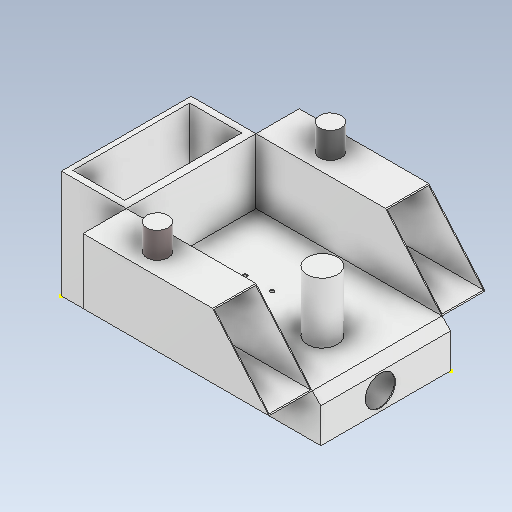
# Autodesk Inventor part: Body
Saved by Autodesk Inventor 2021 (Build 250183000, 183)
## iProperties
Created: 2021-07-15
Part Number: Body
Material: Acetal Resin, White
Document SubType Name: Modeling
Designer: HP
Density: 1.425 g/cm^3
Appearance: Smooth - White
Author: HP
Autodesk Inventor part; units mm, degrees
ref_plane "YZ Plane" through (0, 0, 0) normal (1, 0, 0) x (0, 1, 0)
ref_plane "XZ Plane" through (0, 0, 0) normal (0, 1, 0) x (-1, 0, 0)
sketch "Sketch1" plane through (0, 0, 0) normal (0, 0, 1) x (1, 0, 0)
  line L0 (0, 0) -> (300, 0)
  line L1 (300, 0) -> (300, 50)
  line L2 (300, 50) -> (0, 50)
  line L3 (0, 50) -> (0, 0)
  dimension "d0" = 300
  dimension "d1" = 50
  constraints: 8 end point, 2 parallel, 1 horizontal, 1 perpendicular
  measures "d0" distance of L2.end L1.end
  measures "d1" distance of L0.end L1.end
extrude "Extrusion1" add sketch "Sketch1" along normal blind 150
sketch "Sketch2" plane through (0, 50, 0) normal (0, 1, 0) x (1, 0, 0)
  line L0 (0, 0) -> (0, -150) projected
  line L1 (300, -150) -> (0, -150) projected
  line L2 (0, 0) -> (75, 0)
  line L3 (75, 0) -> (75, -150)
  line L4 (75, -150) -> (0, -150)
  line L5 (0, -150) -> (0, 0)
  line L6 (5.9297, -7.65) -> (65.9297, -7.65)
  line L7 (65.9297, -7.65) -> (65.9297, -142.65)
  line L8 (65.9297, -142.65) -> (5.9297, -142.65)
  line L9 (5.9297, -142.65) -> (5.9297, -7.65)
  dimension "d4" = 75
  dimension "d5" = 60
  dimension "d6" = 135
  dimension "d7" = 7.35
  constraints: 16 end point, 4 parallel, 2 horizontal, 2 perpendicular, 1 point on line
  measures "d4" distance of L3.end L4.end
  measures "d5" distance of L7.end L8.end
  measures "d6" distance of L6.end L7.end
  measures "d7" distance between parallel lines of L8 L1
extrude "Extrusion2" add sketch "Sketch2" along normal blind 75
sketch "Sketch3" plane through (300, 50, 150) normal (0, 1, 0) x (1, 0, 0)
  point P0 (-300, 150)
chamfer "Chamfer1" distance 10 angle 45 1 edges at (300, 50, 75)
sketch "Sketch5" plane through (75, 50, 150) normal (1, 0, 0) x (0, 0, -1)
  point P0 (150, -50)
sketch "Sketch6" plane through (0, 0, 150) normal (0, 0, 1) x (1, 0, 0)
  line L0 (75, 125) -> (224.8279, 125)
  line L1 (290, 50) -> (75, 50) projected
  line L2 (224.8279, 125) -> (290, 50)
  line L3 (75, 125) -> (75, 50)
  line L4 (290, 50) -> (75, 50) projected
  line L5 (75, 50) -> (290, 50)
  point P0 (0, 0)
  constraints: 8 end point, 1 collinear, 1 horizontal
extrude "Extrusion4" add sketch "Sketch6" along normal blind 50
sketch "Sketch7" plane through (0, 0, 150) normal (0, 0, -1) x (-1, 0, 0)
  point P0 (0, 0)
sketch "Sketch8" plane through (0, 0, 0) normal (0, 0, -1) x (-1, 0, 0)
  line L0 (-224.8279, 125) -> (-75, 125) projected
  line L1 (-75, 125) -> (-224.8279, 125)
  line L2 (-290, 50) -> (-300, 40) projected
  line L3 (-224.8279, 125) -> (-290, 50)
  line L4 (-290, 50) -> (-75, 50)
  line L5 (0, 125) -> (-75, 125) projected
  line L6 (-75, 50) -> (-75, 125)
  point P0 (0, 0)
  constraints: 8 end point, 1 collinear, 1 parallel, 1 perpendicular
extrude "Extrusion5" add sketch "Sketch8" along normal blind 50
shell "Shell1" thickness 1 removed faces 2 at (268.276, 75, 183.3333) at (246.5519, 100, -33.3333)
sketch "Sketch9" plane through (75, 125, 150) normal (0, 1, 0) x (1, 0, 0)
  circle A0 centre (61.0187, -25) radius 12.5
  circle A1 centre (61.0187, 175) radius 12.5
  circle A2 centre (61.0187, -29.8112) radius 0.5
  circle A3 centre (61.0187, -24.9762) radius 0.5
  point P0 (-75, 150)
  dimension "d22" = 25
  dimension "d23" = 25
  dimension "d32" = 1
  dimension "d33" = 1
  dimension "d34" = 4.835
  constraints: 4 centre point
  measures "d22" diameter of A0
  measures "d23" diameter of A1
  measures "d32" diameter of A2
  measures "d33" diameter of A3
  measures "d34" distance of A2.centre A3.centre
extrude "Extrusion6" add sketch "Sketch9" along normal blind 30 contours A0 | A1 | A2 | A3
sketch "Sketch10" plane through (75, 50, 150) normal (0, 1, 0) x (1, 0, 0)
  circle A0 centre (165.7607, 60.9468) radius 17.5
  point P0 (-75, 150)
  dimension "d26" = 35
  constraints: 1 centre point
  measures "d26" diameter of A0
extrude "Extrusion7" add sketch "Sketch10" along normal blind 70
sketch "Sketch11" plane through (300, 0, 150) normal (1, 0, 0) x (0, 0, -1)
  point P0 (150, 0)
sketch "Sketch12" plane through (300, 0, 150) normal (1, 0, 0) x (0, 0, -1)
  point P0 (150, 0)
sketch "Sketch13" plane through (300, 0, 150) normal (1, 0, 0) x (0, 0, -1)
  circle A0 centre (68.7762, 20.842) radius 17.5
  point P0 (150, 0)
  dimension "d29" = 35
  constraints: 1 centre point
  measures "d29" diameter of A0
extrude "Extrusion8" cut sketch "Sketch13" against normal blind 5
sketch "Sketch14" plane through (136.0187, 155, 175) normal (0, 1, 0) x (1, 0, 0)
  point P0 (-136.0187, 175)
sketch "Sketch15" plane through (300, 0, 150) normal (1, 0, 0) x (0, 0, -1)
  point P0 (150, 0)
sketch "Sketch16" plane through (75, 50, 150) normal (1, 0, 0) x (0, 0, -1)
  circle A0 centre (48.1445, -35.3763) radius 2.5
  point P0 (150, -50)
  dimension "d35" = 5
  constraints: 1 centre point
  measures "d35" diameter of A0
extrude "Extrusion9" add sketch "Sketch16" along normal blind 200
ref_plane "Work Plane1" through (171.5, 50, 150) normal (1, 0, 0) x (0, 0, -1)
sketch "Sketch18" plane through (75, 50, 150) normal (0, 1, 0) x (1, 0, 0)
  line L0 (0, 50.6445) -> (200, 50.6445) projected
  circle A0 centre (60.705, 37.995) radius 2.5
  circle A1 centre (60.705, 76.6331) radius 2.5
  circle A2 centre (91.9572, 38.2169) radius 2.5
  circle A3 centre (91.9572, 76.6331) radius 2.5
  point P0 (-75, 150)
  dimension "d44" = 5
  dimension "d45" = 5
  constraints: 4 centre point
  measures "d44" diameter of A2
  measures "d45" diameter of A3
extrude "Extrusion11" cut sketch "Sketch18" against normal blind 10
sketch "Sketch19" plane through (75, 50, 150) normal (0, 1, 0) x (1, 0, 0)
  point P0 (-75, 150)
sketch "Sketch20" plane through (75, 50, 150) normal (0, 1, 0) x (1, 0, 0)
  point P0 (-75, 150)
body "Solid1"
